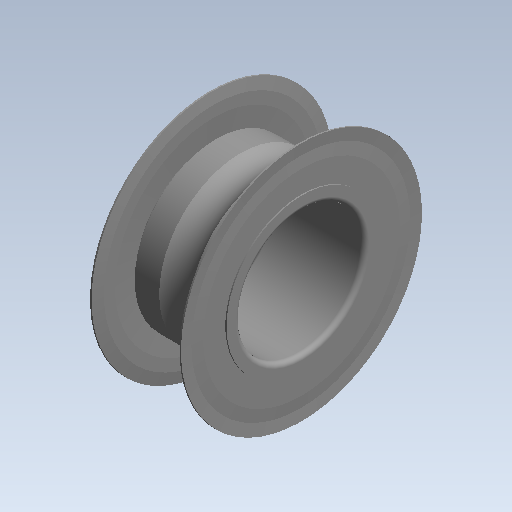
# Autodesk Inventor part: W 619/8 R-2Z_PART1
Saved by Autodesk Inventor 2020 (Build 240168000, 168)
## iProperties
Part Number: W 619/8 R-2Z_PART1
Material: Generic
Catalog Web Link: www.cadenas.de
Description: -Deep groove ball bearings
Vendor: SKF
Document SubType Name: Modeling
Designer: partserver
Manufacturer: SKF
Mass: 0.224222 g
Surface Area: 8.64415 cm^2
Volume: 0.224222 cm^3
Density: 1 g/cm^3
Appearance: PSOLRGB-175-175-175
Category: PARTsolutions
Company: SKF
PSOL_IDENT_0: {$CADENAS_DATA\23d-libs\skf\bearings_units_and_housings\ball_bearings\deep_groove_ball_bearings\bb1_
PSOL_IDENT_1: 001_101.prj},203 {VTYP=3D},{NB=W 619/8 R-2Z_PART1},{LINA=W 619/8 R-2Z_PART1},{NN=BB1_001_101_PART1},
PSOL_IDENT_2: {NOPRJ=TRUE},{DATE=23.12.2020 11:57:27},{GEOMDATE=21.12.2020 15:18:31},{VERSION=},{LINEID=22940},{WB
PSOL_IDENT_3: VAR=},{WBNUMERIC=}  {NB=W 619/8 R-2Z_PART1},{LINA=W 619/8 R-2Z_PART1},{KT=DUMMY},{DESIGNATION=W 619/
PSOL_IDENT_4: 8 R-2Z},{R12=0.30},{DD=8.000},{D=19.000},{B=6.000},{C=},{CX=},{CXX=1.5},{CA=1.500},{XXVARIANT=Flange
PSOL_IDENT_5: d outer ring},{XXDESIGN=Single row stainless steel},{XXSEALING=Shield on both sides},{DESIGN=dgbbwr2
PSOL_IDENT_6: zs},{DESIGNIR=dgbbwr2zs},{VARIANT=Flanged outer ring},{DD1=10.50},{DD2=9.8},{DD2X=},{DD2A=9.80},{D1=
PSOL_IDENT_7: 15.50},{D1X=MIN},{D2=16.66},{D2A=16.66},{D3=22},{D3X=},{D3A=22.000},{D4=},{HH=MIN},{BB=MIN},{BBX=},{
PSOL_IDENT_8: BBA=0.000},{FF=},{R0MAX=MIN},{R0=MIN},{PITCH=13.00},{DW=3.175},{DDAMIN=9.700},{DDAMAX=9.700},{DDBMIN=
PSOL_IDENT_9: MIN},{DDBMAX=MIN},{DBMIN=MIN},{DAMAX=MIN},{BBAMIN=MIN},{CAMAX=MIN},{RAMAX=0.300},{LOAD1=1.250},{LOAD
PSOL_IDENT_10: 2=0.455},{LOAD3=0.020},{SPEED1=85000},{SPEED2=43000},{KR=0.025},{F0=6.600},{Z=7},{II=1},{MASS=0.008}
PSOL_IDENT_11: ,{BEARING=W 619/8 R-2Z},{RING=},{HELP=1.750},{HELP2=1.170},{DD1ALG=5.250},{YALG=5.250},{PITCH1=13.00
PSOL_IDENT_12: 0},{DW1=3.175},{YALG1=7.750},{HALG1=1.750},{SH=4.900},{CU=0.565},{HALG=1.25},{B1=-3.22875},{SHIELDHE
PSOL_IDENT_13: LP=2},{D4A=0.000},{FFA=0.000},{RS1=}
NB: W 619/8 R-2Z_PART1
NT: Deep groove ball bearings
NBSYN: $DESIGNATION._PART1
LINA: W 619/8 R-2Z_PART1
CATALOG: SKF
SUPPLIER: SKF
ARTICLENO: W 619/8 R-2Z_PART1
BOMINFO: W 619/8 R-2Z_PART1
CREATOR: CADENAS GmbH
Title: W 619/8 R-2Z_PART1
Author: Cadenas PARTsolutions
Comments: Deep groove ball bearings
Autodesk Inventor part; units mm, degrees
ref_plane "YZ Plane" through (0, 0, 0) normal (1, 0, 0) x (0, 1, 0)
ref_plane "XZ Plane" through (0, 0, 0) normal (0, 1, 0) x (-1, 0, 0)
ref_plane "XY Plane" through (0, 0, 0) normal (0, 0, 1) x (1, 0, 0)
sketch "Sketch_40" plane through (0, 0, 0) normal (0, 0, 1) x (1, 0, 0)
  line L0 (3, 0) -> (-3, 0)
  line L1 (0, 5.175) -> (0, 4.3)
  arc A0 (0, 4.3) -> (0.3, 4) centre (0.3, 4.3) ccw
  line L2 (0.3, 4) -> (5.7, 4)
  arc A1 (5.7, 4) -> (6, 4.3) centre (5.7, 4.3) ccw
  line L3 (6, 4.3) -> (6, 5.175)
  arc A2 (6, 5.175) -> (5.925, 5.25) centre (5.925, 5.175) ccw
  line L4 (5.925, 5.25) -> (3.9786, 5.25)
  arc A3 (2.0214, 5.25) -> (3.9786, 5.25) centre (3, 6.5) ccw
  line L5 (2.0214, 5.25) -> (0.075, 5.25)
  arc A4 (0.075, 5.25) -> (0, 5.175) centre (0.075, 5.175) ccw
  constraints: 12 end point, 10 point on circle, 5 centre point
revolve "Revolution1" add sketch "Sketch_40" angle 360 about axis through (3, 0, 0) along (1, 0, 0)
sketch "Sketch_42" plane through (0, 0, 0) normal (0, 0, 1) x (1, 0, 0)
  line L0 (3, 0) -> (-3, 0)
  line L1 (0, 11.4) -> (0, 4.9)
  line L2 (0, 4.9) -> (0.15, 4.9)
  arc A0 (0.15, 4.9) -> (0.45, 5.2) centre (0.15, 5.2) ccw
  line L3 (0.45, 5.2) -> (0.45, 11.1)
  line L4 (0.45, 11.1) -> (5.55, 11.1)
  line L5 (5.55, 11.1) -> (5.55, 5.2)
  arc A1 (5.55, 5.2) -> (5.85, 4.9) centre (5.85, 5.2) ccw
  line L6 (5.85, 4.9) -> (6, 4.9)
  line L7 (6, 4.9) -> (6, 11.4)
  line L8 (6, 11.4) -> (0, 11.4)
  constraints: 18 end point, 4 point on circle, 2 centre point
revolve "Revolution2" cut sketch "Sketch_42" angle 360 about axis through (3, 0, 0) along (1, 0, 0)
sketch "Sketch_43" plane through (0, 0, 0) normal (0, 0, 1) x (1, 0, 0)
  line L0 (50, 0) -> (-50, 0)
  line L1 (0.075, 7.75) -> (0.12, 7.0375)
  line L2 (0.12, 7.0375) -> (0.075, 6.325)
  line L3 (0.075, 6.325) -> (0.075, 4.9)
  line L4 (0.075, 4.9) -> (0.165, 4.9)
  line L5 (0.165, 4.9) -> (0.255, 6.325)
  line L6 (0.255, 6.325) -> (0.255, 7.0375)
  line L7 (0.255, 7.0375) -> (0.165, 7.75)
  line L8 (0.165, 7.75) -> (0.075, 7.75)
  constraints: 18 end point
revolve "Revolution3" add sketch "Sketch_43" angle 360 about axis through (50, 0, 0) along (1, 0, 0)
sketch "Sketch_44" plane through (0, 0, 0) normal (0, 0, 1) x (1, 0, 0)
  line L0 (50, 0) -> (-50, 0)
  line L1 (5.745, 7.0375) -> (5.745, 6.325)
  line L2 (5.745, 6.325) -> (5.835, 4.9)
  line L3 (5.835, 4.9) -> (5.925, 4.9)
  line L4 (5.925, 4.9) -> (5.925, 6.325)
  line L5 (5.925, 6.325) -> (5.88, 7.0375)
  line L6 (5.88, 7.0375) -> (5.925, 7.75)
  line L7 (5.925, 7.75) -> (5.835, 7.75)
  line L8 (5.835, 7.75) -> (5.745, 7.0375)
  constraints: 18 end point
revolve "Revolution4" add sketch "Sketch_44" angle 360 about axis through (50, 0, 0) along (1, 0, 0)
body "Solid1"
